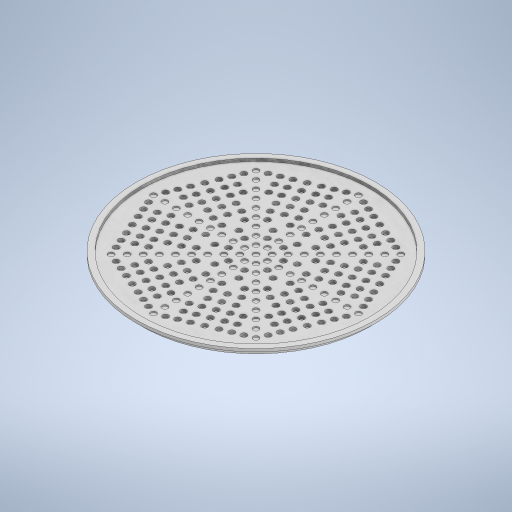
# Autodesk Inventor part: Speaker(H)
Saved by Autodesk Inventor 2023 (Build 270158030, 158C)
## iProperties
Created: 2023-03-05
Part Number: Speaker(H)
Material: Generic
Document SubType Name: Modeling
Designer: mpino
Density: 1 g/cm^3
Appearance: Default
Author: mpino
Autodesk Inventor part; units mm, degrees
ref_plane "YZ Plane" through (0, 0, 0) normal (1, 0, 0) x (0, 1, 0)
ref_plane "XZ Plane" through (0, 0, 0) normal (0, 1, 0) x (-1, 0, 0)
ref_plane "XY Plane" through (0, 0, 0) normal (0, 0, 1) x (1, 0, 0)
sketch "Sketch1" plane through (0, 0, 0) normal (0, 1, 0) x (-1, 0, 0)
  circle A0 centre (0, 0) radius 25.4
  dimension "d0" = 50.8
  constraints: 1 centre point, 1 coincident
  measures "d0" diameter of A0
extrude "Extrusion1" add sketch "Sketch1" along normal blind 1.27
sketch "Sketch2" plane through (0, 1.27, 0) normal (0, 1, 0) x (1, 0, 0)
  circle A0 centre (0, 0) radius 25.4
  circle A1 centre (0, 0) radius 26.67
  dimension "d3" = 50.8
  dimension "d4" = 53.34
  constraints: 2 centre point, 2 coincident
  measures "d3" diameter of A0
  measures "d4" diameter of A1
extrude "Extrusion2" add sketch "Sketch2" along normal blind 0.635
sketch "Sketch3" plane through (0, 0, 0) normal (0, -1, 0) x (1, 0, 0)
  line L0 (-4.7625, 3.175) -> (-7.9375, 3.175)
  line L1 (-7.9375, 3.175) -> (-7.9375, -3.175)
  line L2 (-7.9375, -3.175) -> (-4.7625, -3.175)
  line L3 (-4.7625, -3.175) -> (-4.7625, 3.175)
  line L4 (-4.7625, 3.175) -> (-7.9375, -3.175) construction
  line L5 (-7.9375, 3.175) -> (-4.7625, -3.175) construction
  point P0 (0, 0)
  point P1 (-6.35, 0)
  dimension "d7" = 6.35
  dimension "d8" = 6.35
  dimension "d9" = 3.175
  dimension "d10" = 4.7625
  constraints: 12 end point, 2 midpoint, 2 parallel, 1 horizontal, 1 perpendicular
  measures "d7" distance of point (-6.35, 0) point (0, 0)
  measures "d8" distance of L2.end L0.start
  measures "d9" distance of L0.start L0.end
  measures "d10" distance from line of point (0, 0) L3
extrude "Extrusion3" cut sketch "Sketch3" against normal blind 0.254
sketch "Sketch4" plane through (0, 1.27, 0) normal (0, 1, 0) x (1, 0, 0)
  circle A0 centre (0, 0) radius 0.635
  dimension "d13" = 1.27
  constraints: 1 centre point, 1 coincident
  measures "d13" diameter of A0
extrude "Extrusion4" cut sketch "Sketch4" against normal blind 0.254
pattern_linear "Rectangular Pattern1" count 10 spacing 2.54 along (1, 0, 0) of "Extrusion4"
pattern_circular "Circular Pattern1" count 8 over 360 about axis through (0, 1.27, 0) along (0, 1, 0) of "Extrusion4", "Rectangular Pattern1"
sketch "Sketch5" plane through (0, 1.27, 0) normal (0, 1, 0) x (1, 0, 0)
  circle A0 centre (0, -5.08) radius 0.635 projected
  circle A1 centre (3.5921, -3.5921) radius 0.635 projected
  circle A2 centre (5.3882, -5.3882) radius 0.635 projected
  circle A3 centre (0, -7.62) radius 0.635 projected
  circle A4 centre (0, -10.16) radius 0.635 projected
  circle A5 centre (7.1842, -7.1842) radius 0.635 projected
  circle A6 centre (8.9803, -8.9803) radius 0.635 projected
  circle A7 centre (0, -12.7) radius 0.635 projected
  circle A8 centre (0, -15.24) radius 0.635 projected
  circle A9 centre (0, -17.78) radius 0.635 projected
  circle A10 centre (10.7763, -10.7763) radius 0.635 projected
  circle A11 centre (12.5724, -12.5724) radius 0.635 projected
  circle A12 centre (14.3684, -14.3684) radius 0.635 projected
  circle A13 centre (16.1645, -16.1645) radius 0.635 projected
  circle A14 centre (0, -20.32) radius 0.635 projected
  circle A15 centre (0, -22.86) radius 0.635 projected
  line L0 (0, -5.08) -> (3.5921, -3.5921)
  line L1 (0, -7.62) -> (5.3882, -5.3882)
  line L2 (0, -10.16) -> (7.1842, -7.1842)
  line L3 (0, -12.7) -> (8.9803, -8.9803)
  line L4 (0, -15.24) -> (10.7763, -10.7763)
  line L5 (0, -20.32) -> (14.3684, -14.3684)
  line L6 (0, -17.78) -> (12.5724, -12.5724)
  line L7 (0, -22.86) -> (16.1645, -16.1645)
  circle A16 centre (1.7961, -4.3361) radius 0.635
  line L8 (1.7961, -4.3361) -> (8.0822, -19.5122)
  line L9 (0, -7.62) -> (2.6941, -6.5041)
  circle A17 centre (2.6941, -6.5041) radius 0.635
  line L10 (0, -10.16) -> (3.5921, -8.6721)
  line L11 (3.5921, -8.6721) -> (7.1842, -7.1842)
  circle A18 centre (1.7961, -9.4161) radius 0.635
  circle A19 centre (5.3882, -7.9282) radius 0.635
  line L12 (0, -12.7) -> (4.4901, -10.8401)
  line L13 (8.9803, -8.9803) -> (4.4901, -10.8401)
  circle A20 centre (2.2451, -11.7701) radius 0.635
  circle A21 centre (6.7352, -9.9102) radius 0.635
  circle A22 centre (4.4901, -10.8401) radius 0.635
  line L14 (2.2451, -11.7701) -> (5.8372, -20.4422)
  line L15 (2.2451, -11.7701) -> (11.6317, -11.7701) construction
  line L16 (6.7352, -9.9102) -> (10.3273, -18.5823)
  line L17 (6.7352, -9.9102) -> (16.1218, -9.9102) construction
  circle A23 centre (3.1431, -13.9381) radius 0.635
  circle A24 centre (5.3882, -13.0082) radius 0.635
  circle A25 centre (7.6332, -12.0782) radius 0.635
  circle A26 centre (4.0411, -16.1061) radius 0.635
  circle A27 centre (8.5312, -14.2462) radius 0.635
  circle A28 centre (6.2862, -15.1762) radius 0.635
  circle A29 centre (4.9391, -18.2741) radius 0.635
  circle A30 centre (7.1842, -17.3442) radius 0.635
  circle A31 centre (9.4293, -16.4143) radius 0.635
  line L18 (0, -17.78) -> (4.0411, -16.1061)
  line L19 (8.5312, -14.2462) -> (12.5724, -12.5724)
  circle A32 centre (2.0206, -16.9431) radius 0.635
  circle A33 centre (10.5518, -13.4093) radius 0.635
  line L20 (2.0206, -16.9431) -> (3.8166, -21.2791)
  line L21 (2.0206, -16.9431) -> (6.7139, -16.9431) construction
  line L22 (10.5518, -13.4093) -> (12.3479, -17.7454)
  line L23 (10.5518, -13.4093) -> (15.2451, -13.4093) construction
  circle A34 centre (2.9186, -19.1111) radius 0.635
  circle A35 centre (11.4498, -15.5773) radius 0.635
  circle A36 centre (3.8166, -21.2791) radius 0.635
  circle A37 centre (5.8372, -20.4422) radius 0.635
  circle A38 centre (8.0822, -19.5122) radius 0.635
  circle A39 centre (10.3273, -18.5823) radius 0.635
  circle A40 centre (12.3479, -17.7454) radius 0.635
  line L24 (12.3479, -17.7454) -> (16.1645, -16.1645)
  line L25 (3.8166, -21.2791) -> (0, -22.86)
  circle A41 centre (1.9083, -22.0696) radius 0.635
  circle A42 centre (14.2562, -16.9549) radius 0.635
  point P0 (0, 0)
  dimension "d22" = 1.27
  dimension "d23" = 1.27
  dimension "d24" = 1.27
  dimension "d25" = 1.27
  dimension "d26" = 1.27
  dimension "d27" = 1.27
  dimension "d28" = 1.27
  dimension "d29" = 67.5
  dimension "d30" = 67.5
  dimension "d31" = 1.27
  dimension "d32" = 1.27
  dimension "d33" = 1.27
  dimension "d34" = 1.27
  dimension "d35" = 1.27
  dimension "d36" = 1.27
  dimension "d37" = 1.27
  dimension "d38" = 1.27
  dimension "d39" = 1.27
  dimension "d40" = 1.27
  dimension "d41" = 1.27
  dimension "d42" = 67.5
  dimension "d43" = 67.5
  dimension "d44" = 1.27
  dimension "d45" = 1.27
  dimension "d46" = 1.27
  dimension "d47" = 1.27
  dimension "d48" = 1.27
  dimension "d49" = 1.27
  dimension "d50" = 1.27
  dimension "d51" = 1.27
  dimension "d52" = 1.27
  constraints: 52 end point, 27 centre point, 20 midpoint, 18 point on line, 7 coincident, 4 collinear, 4 equal length, 4 horizontal
  measures "d22" diameter of A16
  measures "d23" diameter of A17
  measures "d24" diameter of A18
  measures "d25" diameter of A19
  measures "d26" diameter of A20
  measures "d27" diameter of A21
  measures "d28" diameter of A22
  measures "d29" angle of L14 L15
  measures "d30" angle of L16 L17
  measures "d31" diameter of A23
  measures "d32" diameter of A24
  measures "d33" diameter of A25
  measures "d34" diameter of A26
  measures "d35" diameter of A27
  measures "d36" diameter of A28
  measures "d37" diameter of A29
  measures "d38" diameter of A30
  measures "d39" diameter of A31
  measures "d40" diameter of A32
  measures "d41" diameter of A33
  measures "d42" angle of L20 L21
  measures "d43" angle of L22 L23
  measures "d44" diameter of A34
  measures "d45" diameter of A35
  measures "d46" diameter of A36
  measures "d47" diameter of A37
  measures "d48" diameter of A38
  measures "d49" diameter of A39
  measures "d50" diameter of A40
  measures "d51" diameter of A41
  measures "d52" diameter of A42
extrude "Extrusion5" cut sketch "Sketch5" against normal blind 0.635 contours A19 L2 | L2 A19 | A42 L7 | L7 A42 | A41 L7 | L7 A41 | A22 L3 L8 | L8 L3 A22 | A18 L2 | L2 A18 | A17 L1 L8 | L8 L1 A17 | A16 L0 | L0 L8 A16 | L0 A16 L8 | L8 A17 L1 | L1 A17 L8 | L8 A22 L3 | L3 A22 L8 | A21 L3 | L3 L16 A21 | A20 L14 L3 | L3 A20 | A24 L4 L8 | L8 L4 A24 | L3 A21 L16 | L14 A20 L3 | L8 A24 L4 | L4 A24 L8 | A25 L4 L16 | L16 L4 A25 | L4 L16 A25 | A23 L14 L4 | L4 L14 A23 | L4 A25 L16 | L14 L4 A23 | A28 L6 L8 | L8 L6 A28 | L14 A23 L4 | L8 A28 L6 | L6 A28 L8 | A27 L6 L16 | L16 L6 A27 | L6 L16 A27 | A26 L14 L6 | L6 L14 A26 | L6 A27 L16 | L14 L6 A26 | A30 L5 L8 | L8 L5 A30 | L14 A26 L6 | A33 L6 | L6 L22 A33 | L8 A30 L5 | L5 A30 L8 | A31 L5 L16 | L16 L5 A31 | L6 A33 L22 | A32 L20 L6 | L6 A32 | L5 L16 A31 | A29 L14 L5 | L5 L14 A29 | L5 A31 L16 | L14 L5 A29 | A35 L5 L22 | L22 L5 A35 | L20 A32 L6 | A38 L7 L8 | L8 L7 A38 | L14 A29 L5 | L5 L22 A35 | L5 A35 L22 | L7 A38 | A39 L7 L16 | L16 L7 A39 | A34 L20 L5 | L5 L20 A34 | L20 L5 A34 | L7 A39 | A37 L7 | L7 L14 A37 | L14 L7 A37 | A40 L7 L22 | L22 L7 A40 | L20 A34 L5 | L7 A40 | A36 L7 | L7 L20 A36 | L20 L7 A36
pattern_circular "Circular Pattern2" count 8 over 360 about axis through (0, 1.27, 0) along (0, 1, 0) of "Extrusion5"
body "Solid1"
